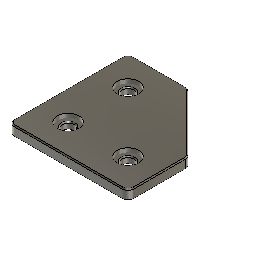
EXTRUSIONbracket (Autodesk Fusion 360 design; units mm, degrees)
Autodesk Fusion 360 part; units mm, degrees
sketch "bracketSketch" plane through (0, 0, 0) normal (0, 0, 1) x (1, 0, 0)
  line L0 (0, 0) -> (60, 0)
  line L1 (60, 0) -> (60, 60)
  line L2 (60, 60) -> (0, 60)
  line L3 (0, 60) -> (0, 0)
  line L4 (0, 15) -> (60, 15) construction
  line L5 (15, 0) -> (15, 60) construction
  line L6 (0, 45) -> (60, 45) construction
  line L7 (45, 0) -> (45, 60) construction
  dimension "d1" = 60
  dimension "d2" = 60
  dimension "d3" = 15
  dimension "d4" = 15
  dimension "d10" = 15
  dimension "d11" = 15
  constraint horizontal L0
  constraint vertical L1
  constraint horizontal L2
  constraint vertical L3
  constraint coincident L0.start L3.end
  constraint coincident L3 L4.start
  constraint coincident L1 L4.end
  constraint perpendicular L1 L4
  constraint coincident L0 L5.start
  constraint coincident L2 L5.end
  constraint perpendicular L2 L5
  constraint coincident L3 L6.start
  constraint coincident L1 L6.end
  constraint perpendicular L1 L6
  constraint coincident L0 L7.start
  constraint coincident L2 L7.end
  constraint perpendicular L2 L7
  measures "d1" distance of L0.start L0.end
  measures "d2" distance of L0.start L2.end
  measures "d3" distance of L0 L4
  measures "d4" distance of L3 L5
  measures "d10" distance of L2 L6
  measures "d11" distance of L1 L7
extrude "Extrude1" add sketch "bracketSketch" along normal blind 5
chamfer "Chamfer4" distance 30 angle 45 1 edges at (60, 60, 2.5)
hole "Hole1" at (15, 15, 5) direction (0, 0, -1) diameter 6 depth 5 tip angle 180 counterbore diameter 11 counterbore depth 2
chamfer "Chamfer3" distance 0.5 angle 45 1 edges at (12.203, 16.0848, 3)
pattern_linear "R-Pattern1" count 2 spacing 30 along (0, 1, 0) of "Hole1", "Chamfer3"
pattern_linear "R-Pattern2" count 2 spacing 30 along (1, 0, 0) of "Hole1", "Chamfer3"
fillet "Fillet2" radius 3 5 edges at (60, 0, 2.5) (0, 60, 2.5) (0, 0, 2.5) (60, 30, 2.5) (30, 60, 2.5)
chamfer "Chamfer5" distance 0.5 angle 45 20 edges at (0, 30, 5) (0.8787, 0.8787, 5) (30, 0, 5) (59.1213, 0.8787, 5) (60, 15.8787, 5) (59.7716, 29.9054, 5) (45, 45, 5) (29.9054, 59.7716, 5) (15.8787, 60, 5) (0.8787, 59.1213, 5) (59.1213, 0.8787, 0) (60, 15.8787, 0) (59.7716, 29.9054, 0) (45, 45, 0) (29.9054, 59.7716, 0) (15.8787, 60, 0) (0.8787, 59.1213, 0) (0, 30, 0) (0.8787, 0.8787, 0) (30, 0, 0)
